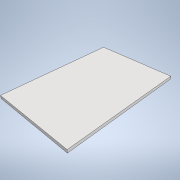
# Autodesk Inventor part: ChairTop
Saved by Autodesk Inventor 2022 (Build 260153000, 153)
## iProperties
Created: 2021-12-19
Part Number: ChairTop
Material: Generic
Document SubType Name: Modeling
Designer: dangl
Density: 1 g/cm^3
Appearance: Default
Author: dangl
Autodesk Inventor part; units mm, degrees
ref_plane "YZ Plane" through (0, 0, 0) normal (1, 0, 0) x (0, 1, 0)
ref_plane "XZ Plane" through (0, 0, 0) normal (0, 1, 0) x (-1, 0, 0)
ref_plane "XY Plane" through (0, 0, 0) normal (0, 0, 1) x (1, 0, 0)
sketch "Sketch1" plane through (0, 0, 0) normal (0, 1, 0) x (-1, 0, 0)
  line L0 (5, 7.5) -> (-5, 7.5)
  line L1 (-5, 7.5) -> (-5, -7.5)
  line L2 (-5, -7.5) -> (5, -7.5)
  line L3 (5, -7.5) -> (5, 7.5)
  point P0 (0, 0)
  dimension "d0" = 15
  dimension "d1" = 10
  dimension "d2" = 5
  dimension "d3" = 7.5
  constraints: 8 end point, 2 parallel, 1 horizontal, 1 perpendicular
  measures "d0" distance of L2.end L0.start
  measures "d1" distance of L1.end L2.end
  measures "d2" distance from line of point (0, 0) L3
  measures "d3" distance from line of point (0, 0) L2
extrude "Extrusion1" add sketch "Sketch1" along normal blind 1.2
sketch "Sketch2" plane through (5, 0, 7.5) normal (1, 0, 0) x (0, 0, -1)
  line L0 (0, 0) -> (0, 1.2) projected
  line L1 (0, 0) -> (0, 0.8)
  line L2 (0, 0.8) -> (1.3856, 0)
  line L3 (0, 0) -> (15, 0) projected
  line L4 (0, 0) -> (1.3856, 0)
  line L5 (7.5, 0) -> (7.5, 5.1118)
  line L6 (15, 0) -> (15, 1.2)
  line L7 (15, 0) -> (15, 0.8)
  line L8 (15, 0.8) -> (13.6144, 0)
  line L9 (15, 0) -> (13.6144, 0)
  dimension "d6" = 0.8
  dimension "d7" = 30
  constraints: 16 end point, 3 point on line, 3 symmetric about line, 1 perpendicular, 1 vertical
  measures "d6" distance of L0.start L1.end
  measures "d7" angle of L3 L2
extrude "Extrusion2" cut sketch "Sketch2" against normal through all
sketch "Sketch3" plane through (-5, 1.2, 7.5) normal (0, 0, 1) x (1, 0, 0)
  line L0 (0, -1.2) -> (0, -0.4) projected
  line L1 (0, -0.4) -> (0, -1.2)
  line L2 (0, -1.2) -> (1.3856, -1.2)
  line L3 (10, -1.2) -> (0, -1.2) projected
  line L4 (0, -0.4) -> (1.3856, -1.2)
  line L5 (5, -1.2) -> (5, 0.9136)
  line L6 (10, -1.2) -> (10, -0.4)
  line L7 (10, -0.4) -> (10, -1.2)
  line L8 (10, -1.2) -> (8.6144, -1.2)
  line L9 (10, -0.4) -> (8.6144, -1.2)
  dimension "d10" = 30
  constraints: 16 end point, 2 symmetric about line, 1 collinear, 1 point on line, 1 vertical
  measures "d10" angle of L2 L4
extrude "Extrusion3" cut sketch "Sketch3" against normal through all
equation "\"d2\" = 0.5 * d1"
equation "\"d3\" = 0.5 * d0"
body "Solid1"
